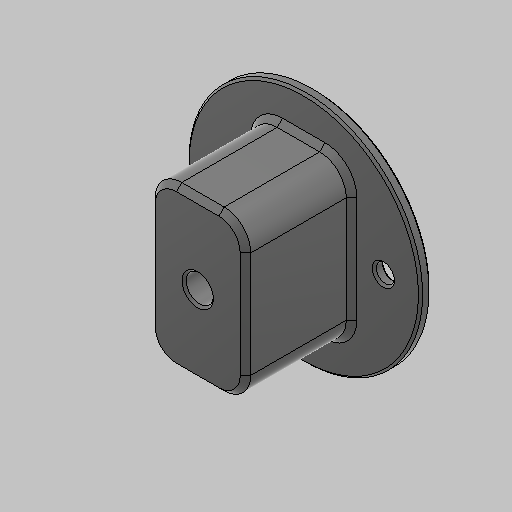
# Autodesk Inventor part: takumar-slit-led
Saved by Autodesk Inventor 2026 (Build 300175050, 175E)
## iProperties
Created: 2025-11-08
Part Number: takumar-slit-led
Material: ABS Plastic
Document SubType Name: Modeling
Designer: queezz
Density: 1.06 g/cm^3
Appearance: Smooth - Black
Author: queezz
Autodesk Inventor part; units mm, degrees
ref_plane "YZ Plane" through (0, 0, 0) normal (1, 0, 0) x (0, 1, 0)
ref_plane "XZ Plane" through (0, 0, 0) normal (0, 1, 0) x (-1, 0, 0)
ref_plane "XY Plane" through (0, 0, 0) normal (0, 0, 1) x (1, 0, 0)
sketch "Sketch1" plane through (0, 0, 0) normal (0, 0, 1) x (1, 0, 0)
  circle A0 centre (0, 0) radius 22
  dimension "d0" = 44
  constraints: 1 centre point, 1 coincident
  measures "d0" diameter of A0
extrude "Extrusion1" add sketch "Sketch1" along normal blind 2
sketch "Sketch2" plane through (0, 0, 2) normal (0, 0, 1) x (1, 0, 0)
  line L0 (-15, 0) -> (15, 0) construction
  point P0 (0, 0)
  point P1 (0, 0)
  dimension "d3" = 30
  constraints: 3 coincident, 2 end point, 1 horizontal, 1 midpoint
  measures "d3" distance of L0.start L0.end
hole "Hole1" at (-15, 0, 2) at (15, 0, 2) direction (0, 0, -1) diameter 3.4 end through all
sketch "Sketch3" plane through (0, 0, 2) normal (0, 0, 1) x (1, 0, 0)
  line L0 (-9, 15) -> (9, 15)
  line L1 (9, 15) -> (9, -15)
  line L2 (9, -15) -> (-9, -15)
  line L3 (-9, -15) -> (-9, 15)
  line L4 (7.2, 13.2) -> (-7.2, 13.2)
  line L5 (-7.2, 13.2) -> (-7.2, -13.2)
  line L6 (-7.2, -13.2) -> (7.2, -13.2)
  line L7 (7.2, -13.2) -> (7.2, 13.2)
  point P0 (0, 0)
  point P1 (9, 0)
  point P2 (0, 15)
  dimension "d11" = 30
  dimension "d12" = 18
  dimension "d13" = 1.8
  constraints: 16 end point, 4 parallel, 2 midpoint, 2 perpendicular, 1 horizontal, 1 horizontal alignment, 1 vertical alignment, 3 other
  measures "d11" distance of L0.end L1.end
  measures "d12" distance of L0.start L0.end
  measures "d13" distance between parallel lines of L0 L4
extrude "Extrusion2" cut sketch "Sketch3" against normal blind 2 contours L7 L6 L5 L4
extrude "Extrusion3" add sketch "Sketch3" along normal blind 20
sketch "Sketch4" plane through (0, 0, 22) normal (0, 0, 1) x (1, 0, 0)
  line L0 (-9, -15) -> (9, -15) projected
  line L1 (9, -15) -> (9, 15) projected
  line L2 (9, 15) -> (-9, 15) projected
  line L3 (-9, 15) -> (-9, -15) projected
  line L4 (7.2, 13.2) -> (7.2, -13.2) projected
  line L5 (7.2, -13.2) -> (-7.2, -13.2) projected
  line L6 (-7.2, -13.2) -> (-7.2, 13.2) projected
  line L7 (-7.2, 13.2) -> (7.2, 13.2) projected
  point P0 (0, 0)
extrude "Extrusion4" add sketch "Sketch4" against normal blind 5 contours L4 L5 L6 L7
sketch "Sketch5" plane through (0, 0, 22) normal (0, 0, 1) x (1, 0, 0)
  point P0 (0, 0)
  point P1 (0, 0)
  constraints: 1 coincident
hole "Hole2" at (0, 0, 22) direction (0, 0, -1) diameter 5.1 end through all
fillet "Fillet1" radius 5 8 edges at (-7.2, -13.2, 8.5) (7.2, -13.2, 8.5) (-7.2, 13.2, 8.5) (7.2, 13.2, 8.5) (9, 15, 12) (-9, 15, 12) (-9, -15, 12) (9, -15, 12)
chamfer "Chamfer1" distance 5 angle 45 8 edges at (0, 13.2, 17) (-5.7355, 11.7355, 17) (-7.2, 0, 17) (-5.7355, -11.7355, 17) (0, -13.2, 17) (5.7355, -11.7355, 17) (7.2, 0, 17) (5.7355, 11.7355, 17)
chamfer "Chamfer2" distance 1 angle 45 24 edges at (0, 15, 22) (-7.5355, 13.5355, 22) (-9, 0, 22) (-7.5355, -13.5355, 22) (0, -15, 22) (7.5355, -13.5355, 22) (9, 0, 22) (7.5355, 13.5355, 22) (9, 0, 2) (7.5355, -13.5355, 2) (0, -15, 2) (-7.5355, -13.5355, 2) (-9, 0, 2) (-7.5355, 13.5355, 2) (0, 15, 2) (7.5355, 13.5355, 2) (7.2, 0, 0) (5.7355, 11.7355, 0) (0, 13.2, 0) (-5.7355, 11.7355, 0) (-7.2, 0, 0) (-5.7355, -11.7355, 0) (0, -13.2, 0) (5.7355, -11.7355, 0)
chamfer "Chamfer3" distance 0.4 angle 45 7 edges at (-22, 0, 2) (-22, 0, 0) (15, 1.7, 2) (-15, 1.7, 2) (-15, 1.7, 0) (15, 1.7, 0) (0, 2.55, 22)
body "Solid1"
